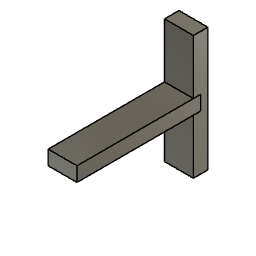
Housing Joint (Autodesk Fusion 360 design; units mm, degrees)
Autodesk Fusion 360 part; units mm, degrees
sketch "Base" plane through (0, 0, 0) normal (0, 0, 1) x (1, 0, 0)
  line L0 (35, 17.5) -> (-35, 17.5)
  line L1 (-35, 17.5) -> (-35, -17.5)
  line L2 (-35, -17.5) -> (35, -17.5)
  line L3 (35, -17.5) -> (35, 17.5)
  line L4 (35, 17.5) -> (-35, -17.5) construction
  line L5 (-35, 17.5) -> (35, -17.5) construction
  dimension "d1" = 70
  dimension "d2" = 35
  constraint horizontal L0
  constraint perpendicular L0 L1
  constraint parallel L0 L2
  constraint parallel L1 L3
  constraint coincident L4 origin
  constraint coincident L5 origin
  measures "d1" distance of L1.end L2.end
  measures "d2" distance of L0.end L1.end
extrude "Extrude1" add sketch "Base" along normal blind 300 makes body 1
sketch "Cut" plane through (0, -17.5, 0) normal (0, -1, 0) x (1, 0, 0)
  line L0 (-35, 0) -> (35, 0)
  line L1 (35, 0) -> (35, 300)
  line L2 (35, 300) -> (-35, 300)
  line L3 (-35, 300) -> (-35, 0)
  line L4 (-35, 167.5) -> (35, 167.5)
  line L5 (35, 167.5) -> (35, 132.5)
  line L6 (35, 132.5) -> (-35, 132.5)
  line L7 (-35, 132.5) -> (-35, 167.5)
  dimension "d5" = 70
  dimension "d6" = 35
  constraint horizontal L4
  constraint vertical L5
  constraint horizontal L6
  constraint vertical L7
  constraint midpoint L1 L5
  measures "d5" distance of L4.start L4.end
  measures "d6" distance of L4.start L6.end
extrude "Extrude2" cut sketch "Cut" against normal blind 17.5 contours L1 L3 L4 L5 L6 L7 bodies 1
sketch "Horizontal Piece" plane through (0, 0, 0) normal (0, -1, 0) x (1, 0, 0)
  line L0 (-35, 132.5) -> (35, 132.5)
  line L1 (35, 132.5) -> (35, 167.5)
  line L2 (35, 167.5) -> (-35, 167.5)
  line L3 (-35, 167.5) -> (-35, 132.5)
  line L4 (-35, 167.5) -> (35, 167.5)
  line L5 (35, 167.5) -> (35, 132.5)
  line L6 (35, 132.5) -> (-35, 132.5)
  line L7 (-35, 132.5) -> (-35, 167.5)
  constraint horizontal L4
  constraint vertical L5
  constraint horizontal L6
  constraint vertical L7
  constraint coincident L0.end L1.start
  constraint coincident L2.end L3.start
extrude "Extrude1'" add sketch "Horizontal Piece" along normal blind 300 separate body makes body 2 in component "Horizontal Piece"
copy_body "Body->Comp1" bodies 1 removing the originals makes body 3 in component "Vertical Piece"
component "Horizontal Piece" placed x (1, 0, 0) y (0, 1, 0) z (0, 0, 1) at (0, 0, 0)
component "Vertical Piece" placed x (1, 0, 0) y (0, 1, 0) z (0, 0, 1) at (0, 0, 0)
equation "d7 = ( -35 / 2 ) * 1 mm"
named bodies: "Horizontal Piece", "Vertical Piece"
